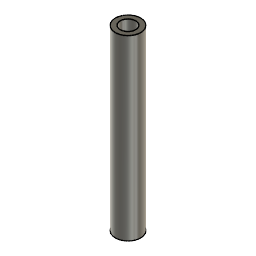
Support (Autodesk Fusion 360 design; units mm, degrees)
part number: 2026-06-24-14-55-54-877
Autodesk Fusion 360 part; units mm, degrees
sketch "Sketch1" plane through (0, 0, 0) normal (0, 0, 1) x (1, 0, 0)
  circle A0 centre (0, 0) radius 2.5
  dimension "d1" = 5
  constraint coincident A0.centre origin
  measures "d1" diameter of A0
extrude "Extrude1" add sketch "Sketch1" along normal blind 35
sketch "Sketch2" plane through (0, 0, 35) normal (0, 0, 1) x (-1, 0, 0)
  circle A0 centre (0, 0) radius 2.5
  constraint coincident A0.centre origin
sketch "Sketch3" plane through (0, 0, 0) normal (0, 0, -1) x (1, 0, 0)
  circle A0 centre (0, 0) radius 2.5
  constraint coincident A0.centre origin
hole "Hole1" at (0, 0, 35) direction (0, 0, -1) diameter 3.05 depth 8 tip angle 180
hole "Hole2" at (0, 0, 0) direction (0, 0, 1) diameter 3.05 depth 8 tip angle 180
